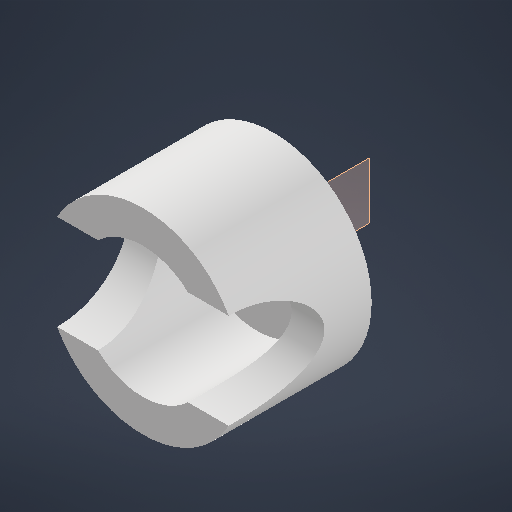
# Autodesk Inventor part: Launchpad
Saved by Autodesk Inventor 2026.1 (Build 301233020, 233B)
## iProperties
Created: 2025-10-09
Part Number: Launchpad
Material: Generic
Document SubType Name: Modeling
Designer: kcosp
Density: 1 g/cm^3
Appearance: Default
Author: kcosp
Autodesk Inventor part; units mm, degrees
ref_plane "YZ Plane" through (0, 0, 0) normal (1, 0, 0) x (0, 1, 0)
ref_plane "XZ Plane" through (0, 0, 0) normal (0, 1, 0) x (-1, 0, 0)
ref_plane "XY Plane" through (0, 0, 0) normal (0, 0, 1) x (1, 0, 0)
sketch "Sketch1" plane through (0, 0, 0) normal (0, 0, 1) x (1, 0, 0)
  circle A0 centre (0, 0) radius 38.1824
  constraints: 1 centre point, 1 coincident
extrude "Extrusion1" add sketch "Sketch1" along normal blind 50.8
sketch "Sketch2" plane through (0, 0, 0) normal (0, 0, -1) x (-1, 0, 0)
  line L0 (-10.125, -10.125) -> (10.125, -10.125) projected
  line L1 (-10.125, 10.125) -> (-10.125, -10.125) projected
  line L2 (10.125, 10.125) -> (-10.125, 10.125) projected
  line L3 (10.125, -10.125) -> (10.125, 10.125) projected
  circle A0 centre (0, 0) radius 25.4 projected
  circle A1 centre (0, 0) radius 25.5
  dimension "d22" = 51
  dimension "d23" = 50.8
  constraints: 1 centre point, 1 coincident
  measures "d22" diameter of A1
  measures "d23" diameter of A0
extrude "Extrusion2" cut sketch "Sketch2" against normal blind 5 contours L1 L2 L3 L0 | A0 | A1
sketch "Sketch4" plane through (0, 0, 50.8) normal (0, 0, 1) x (1, 0, 0)
  circle A0 centre (0, 0) radius 25.5 projected
  circle A1 centre (0, 0) radius 25.5
  constraints: 1 centre point, 1 coincident, 1 concentric
extrude "Extrusion4" cut sketch "Sketch4" against normal blind 44.45
ref_plane "Work Plane1" through (0, 10, -2.54) normal (1, 0, 0) x (0, -1, 0)
sketch "Sketch5" plane through (0, 10, -2.54) normal (1, 0, 0) x (0, -1, 0)
  line L0 (-28.1824, -53.34) -> (48.1824, -53.34) projected
  ellipse E0 centre (10, -53.34) end of major axis (28.5443, -53.34) minor radius 32.3873 (28.5443, -53.34) -> (-8.5443, -53.34) ccw
  point P0 (10, -2.54)
  constraints: 2 point on line, 1 midpoint, 4 other
extrude "Extrusion5" cut sketch "Sketch5" along normal through all both and the other way through all
sketch "Sketch6" plane through (0, 10, -2.54) normal (1, 0, 0) x (0, -1, 0)
  point P0 (10, -2.54)
sketch "Sketch7" plane through (0, 0, 6.35) normal (0, 0, 1) x (1, 0, 0)
  circle A0 centre (0, 0) radius 3.975 projected
  circle A1 centre (0, 0) radius 4.1
  dimension "d12" = 8.2
  constraints: 1 centre point, 1 coincident
  measures "d12" diameter of A1
extrude "Extrusion6" cut sketch "Sketch7" against normal blind 10 contours A0 | A1
sketch "Sketch8" plane through (0, 0, 0) normal (0, 0, -1) x (-1, 0, 0)
  circle A0 centre (0, 0) radius 25.4 projected
  line L0 (-17.5031, 18.5443) -> (-33.3767, 18.5443) projected
  line L1 (-33.3767, -18.5443) -> (-17.5031, -18.5443) projected
  line L2 (17.5031, -18.5443) -> (33.3767, -18.5443) projected
  line L3 (33.3767, 18.5443) -> (17.5031, 18.5443) projected
  circle A1 centre (0, 31.8008) radius 3.4055
  circle A2 centre (-15.9004, 27.5403) radius 3.4055
  circle A3 centre (-27.5403, 15.9004) radius 3.4055
  circle A4 centre (-31.8008, 0) radius 3.4055
  circle A5 centre (-27.5403, -15.9004) radius 3.4055
  circle A6 centre (-15.9004, -27.5403) radius 3.4055
  circle A7 centre (0, -31.8008) radius 3.4055
  circle A8 centre (15.9004, -27.5403) radius 3.4055
  circle A9 centre (27.5403, -15.9004) radius 3.4055
  circle A10 centre (31.8008, 0) radius 3.4055
  circle A11 centre (27.5403, 15.9004) radius 3.4055
  circle A12 centre (15.9004, 27.5403) radius 3.4055
  dimension "d15" = 6.811
  dimension "d18" = 360
  constraints: 12 centre point, 25 other
  measures "d15" diameter of A1
sketch "Sketch9" plane through (0, 0, 0) normal (0, 0, -1) x (-1, 0, 0)
  circle A0 centre (0, 31.8008) radius 3.4055 projected
  circle A1 centre (15.9004, 27.5403) radius 3.4055 projected
  circle A2 centre (-15.9004, 27.5403) radius 3.4055 projected
  circle A3 centre (-15.9004, -27.5403) radius 3.4055 projected
  circle A4 centre (0, -31.8008) radius 3.4055 projected
  circle A5 centre (15.9004, -27.5403) radius 3.4055 projected
  circle A6 centre (0, 31.8008) radius 3.4055
  circle A7 centre (15.9004, 27.5403) radius 3.4055
  circle A8 centre (-15.9004, 27.5403) radius 3.4055
  circle A9 centre (-15.9004, -27.5403) radius 3.4055
  circle A10 centre (0, -31.8008) radius 3.4055
  circle A11 centre (15.9004, -27.5403) radius 3.4055
  point P0 (0, 0)
  constraints: 6 centre point, 6 coincident, 6 concentric
extrude "Extrusion7" cut sketch "Sketch8" against normal blind 48 contours A1 | A2 | A6 | A7 | A8 | A12
body "Solid1"
